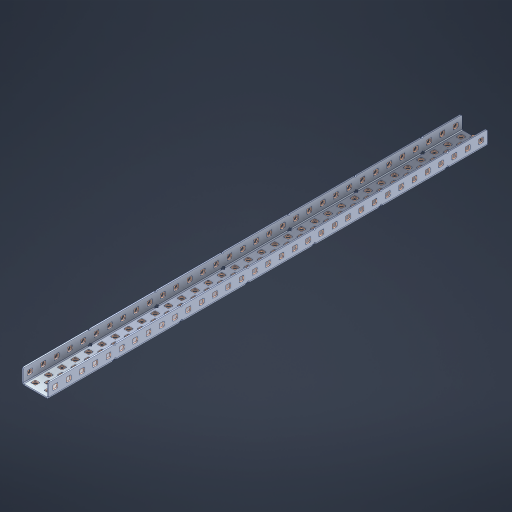
# Autodesk Inventor part: Alu C 1x2x1x35
Saved by Autodesk Inventor 2023 (Build 270158000, 158)
## iProperties
Created: 2022-07-28
Part Number: Alu C 1x2x1x35
Material: Generic
Document SubType Name: Sheet Metal
Designer: ylu12
Density: 1 g/cm^3
Sheet Metal Rule: Default
Appearance: Steel
Author: ylu12
Autodesk Inventor part; units mm, degrees
ref_plane "YZ Plane" through (0, 0, 0) normal (1, 0, 0) x (0, 1, 0)
ref_plane "XZ Plane" through (0, 0, 0) normal (0, 1, 0) x (-1, 0, 0)
sketch "Sketch1" plane through (0, 0, 0) normal (0, 1, 0) x (-1, 0, 0)
  line L0 (-12.7, 0) -> (12.7, 0)
  line L1 (12.7, 0) -> (12.7, -419.1)
  line L2 (12.7, -419.1) -> (-12.7, -419.1)
  line L3 (-12.7, -419.1) -> (-12.7, 0)
  line L4 (12.7, 0) -> (-12.7, -419.1) construction
  point P0 (0, 0)
  point P1 (0, 0)
  dimension "d0" = 25.4
  dimension "d1" = 419.1
  measures "d0" distance of L1.end L2.end
  measures "d1" distance of L0.end L1.end
extrude "Plate1" add sketch "Sketch1" along normal blind 1.1906
sketch "Sketch2" plane through (11.5094, 0, -419.1) normal (1, 0, 0) x (0, 1, 0)
  line L0 (0, 419.1) -> (0, 0)
  line L1 (0, 0) -> (13.8906, 0)
  line L2 (13.8906, 0) -> (13.8906, 419.1)
  line L3 (13.8906, 419.1) -> (0, 419.1)
  constraints: 6 end point, 1 horizontal, 1 perpendicular, 1 vertical
edge flange "Flanges" height 12.7 angle 90 thickness 1.1906 bend radius 0.7937 thickness toward (1, 0, 0) relief tear relief width 1.1906 relief depth 0.5953 corner gap 1.1906 corner form 0 edges at (12.7, 1.1906, -209.55) (-12.7, 1.1906, -209.55) wall of the first edge with corners at (11.5094, 0, 0) (11.5094, 0, -419.1) (11.5094, 13.8906, -419.1) (11.5094, 13.8906, 0)
bend "Bend1"
corner "Corner1"
sketch "Sketch3" plane through (12.7, 1.9844, -419.1) normal (1, 0, 0) x (0, 0, -1)
  line L0 (-414.5534, 7.8676) -> (-410.9466, 7.8676)
  line L1 (-410.4386, 7.3596) -> (-410.4386, 3.7528)
  line L2 (-410.9466, 3.2448) -> (-414.5534, 3.2448)
  line L3 (-415.0614, 3.7528) -> (-415.0614, 7.3596)
  arc A0 (-414.5534, 7.8676) -> (-415.0614, 7.3596) centre (-414.5534, 7.3596) ccw
  arc A1 (-410.4386, 7.3596) -> (-410.9466, 7.8676) centre (-410.9466, 7.3596) ccw
  arc A2 (-410.9466, 3.2448) -> (-410.4386, 3.7528) centre (-410.9466, 3.7528) ccw
  arc A3 (-415.0614, 3.7528) -> (-414.5534, 3.2448) centre (-414.5534, 3.7528) ccw
  line L4 (-419.1, 0) -> (-419.1, 11.9062) construction
  line L5 (-419.1, 11.9062) -> (0, 11.9062) construction
  line L6 (-414.5534, 7.3596) -> (-410.9466, 3.7528) construction
  point P0 (-419.1, -1.9844)
  point P1 (-410.4386, 3.2448)
  point P2 (-415.0614, 3.2448)
  point P3 (-412.75, 5.5562)
  dimension "d16" = 4.6228
  dimension "d17" = 0.508
  dimension "d20" = 6.35
  dimension "d21" = 6.35
  constraints: 10 end point, 8 point on circle, 8 tangent, 4 centre point, 4 point on line, 3 equal radius, 2 parallel, 2 perpendicular, 1 horizontal, 1 midpoint
  measures "d16" distance of point (-410.439, 3.245) point (-415.061, 3.245)
  measures "d17" radius of A0
  measures "d20" distance from line of point (-412.75, 5.556) L4
  measures "d21" distance from line of L5 point (-412.75, 5.556)
extrude "Flange Stamp" cut sketch "Sketch3" against normal blind 1.1906
sketch "Sketch7" plane through (12.7, 1.9844, 0) normal (1, 0, 0) x (0, 0, -1)
  arc A0 (4.5466, 7.8676) -> (4.0386, 7.3596) centre (4.5466, 7.3596) ccw construction
  arc A1 (8.1534, 3.2448) -> (8.6614, 3.7528) centre (8.1534, 3.7528) ccw construction
  circle A2 centre (6.35, 5.5563) radius 2.1844
  line L0 (4.5466, 7.3596) -> (8.1534, 3.7528) construction
  point P0 (0, -1.9844)
  dimension "d46" = 4.3688
  constraints: 2 end point, 1 centre point, 1 midpoint
  measures "d46" diameter of A2
surface extrude "Flange Circle" sketch "Sketch7" against normal up to surface (1.1906 mm away) shown yes curves A2
ref_plane "Flange Pattern Plane" through (12.7, 7.5406, -4.5466) normal (0, 1, 0) x (1, 0, 0)
sketch "Flange Pattern Sketch" plane through (12.7, 7.5406, -4.5466) normal (0, 1, 0) x (1, 0, 0)
  line L0 (0, 3.6068) -> (0, 0) construction
  line L1 (-30.5622, -4.5466) -> (5.5732, -4.5466) construction
  line L2 (0, 0) -> (-1.1906, 0) construction
  point P0 (-12.7, -4.5466)
  point P1 (0, 1.8034)
  point P2 (0, 14.5034)
  point P3 (0, 27.2034)
  point P4 (0, 39.9034)
  point P5 (0, 52.6034)
  point P6 (0, 65.3034)
  point P7 (0, 78.0034)
  point P8 (0, 90.7034)
  point P9 (0, 103.4034)
  point P10 (0, 116.1034)
  point P11 (0, 128.8034)
  point P12 (0, 141.5034)
  point P13 (0, 154.2034)
  point P14 (0, 166.9034)
  point P15 (0, 179.6034)
  point P16 (0, 192.3034)
  point P17 (0, 205.0034)
  point P18 (0, 217.7034)
  point P19 (0, 230.4034)
  point P20 (0, 243.1034)
  point P21 (0, 255.8034)
  point P22 (0, 268.5034)
  point P23 (0, 281.2034)
  point P24 (0, 293.9034)
  point P25 (0, 306.6034)
  point P26 (0, 319.3034)
  point P27 (0, 332.0034)
  point P28 (0, 344.7034)
  point P29 (0, 357.4034)
  point P30 (0, 370.1034)
  point P31 (0, 382.8034)
  point P32 (0, 395.5034)
  point P33 (0, 408.2034)
  point P34 (-25.4, 1.8034)
  point P35 (-25.4, 14.5034)
  point P36 (-25.4, 27.2034)
  point P37 (-25.4, 39.9034)
  point P38 (-25.4, 52.6034)
  point P39 (-25.4, 65.3034)
  point P40 (-25.4, 78.0034)
  point P41 (-25.4, 90.7034)
  point P42 (-25.4, 103.4034)
  point P43 (-25.4, 116.1034)
  point P44 (-25.4, 128.8034)
  point P45 (-25.4, 141.5034)
  point P46 (-25.4, 154.2034)
  point P47 (-25.4, 166.9034)
  point P48 (-25.4, 179.6034)
  point P49 (-25.4, 192.3034)
  point P50 (-25.4, 205.0034)
  point P51 (-25.4, 217.7034)
  point P52 (-25.4, 230.4034)
  point P53 (-25.4, 243.1034)
  point P54 (-25.4, 255.8034)
  point P55 (-25.4, 268.5034)
  point P56 (-25.4, 281.2034)
  point P57 (-25.4, 293.9034)
  point P58 (-25.4, 306.6034)
  point P59 (-25.4, 319.3034)
  point P60 (-25.4, 332.0034)
  point P61 (-25.4, 344.7034)
  point P62 (-25.4, 357.4034)
  point P63 (-25.4, 370.1034)
  point P64 (-25.4, 382.8034)
  point P65 (-25.4, 395.5034)
  point P66 (-25.4, 408.2034)
  dimension "d43" = 25.4
  dimension "d40" = 12.7
  constraints: 1 horizontal, 1 midpoint, 1 vertical, 65 other
  measures "d40" distance of point (0, 1.803) point (0, 14.503)
pattern_sketch "Flange Pattern" of "Flange Circle", "Flange Stamp" from (12.7, 7.5406, -6.35) facing (1, 0, 0) copies at (12.7, 7.5406, -19.05) facing (1, 0, 0) at (12.7, 7.5406, -31.75) facing (1, 0, 0) at (12.7, 7.5406, -44.45) facing (1, 0, 0) at (12.7, 7.5406, -57.15) facing (1, 0, 0) at (12.7, 7.5406, -69.85) facing (1, 0, 0) at (12.7, 7.5406, -82.55) facing (1, 0, 0) at (12.7, 7.5406, -95.25) facing (1, 0, 0) at (12.7, 7.5406, -107.95) facing (1, 0, 0) at (12.7, 7.5406, -120.65) facing (1, 0, 0) at (12.7, 7.5406, -133.35) facing (1, 0, 0) at (12.7, 7.5406, -146.05) facing (1, 0, 0) at (12.7, 7.5406, -158.75) facing (1, 0, 0) at (12.7, 7.5406, -171.45) facing (1, 0, 0) at (12.7, 7.5406, -184.15) facing (1, 0, 0) at (12.7, 7.5406, -196.85) facing (1, 0, 0) at (12.7, 7.5406, -209.55) facing (1, 0, 0) at (12.7, 7.5406, -222.25) facing (1, 0, 0) at (12.7, 7.5406, -234.95) facing (1, 0, 0) at (12.7, 7.5406, -247.65) facing (1, 0, 0) at (12.7, 7.5406, -260.35) facing (1, 0, 0) at (12.7, 7.5406, -273.05) facing (1, 0, 0) at (12.7, 7.5406, -285.75) facing (1, 0, 0) at (12.7, 7.5406, -298.45) facing (1, 0, 0) at (12.7, 7.5406, -311.15) facing (1, 0, 0) at (12.7, 7.5406, -323.85) facing (1, 0, 0) at (12.7, 7.5406, -336.55) facing (1, 0, 0) at (12.7, 7.5406, -349.25) facing (1, 0, 0) at (12.7, 7.5406, -361.95) facing (1, 0, 0) at (12.7, 7.5406, -374.65) facing (1, 0, 0) at (12.7, 7.5406, -387.35) facing (1, 0, 0) at (12.7, 7.5406, -400.05) facing (1, 0, 0) at (12.7, 7.5406, -412.75) facing (1, 0, 0) at (-12.7, 7.5406, -6.35) facing (-1, 0, 0) at (-12.7, 7.5406, -19.05) facing (-1, 0, 0) at (-12.7, 7.5406, -31.75) facing (-1, 0, 0) at (-12.7, 7.5406, -44.45) facing (-1, 0, 0) at (-12.7, 7.5406, -57.15) facing (-1, 0, 0) at (-12.7, 7.5406, -69.85) facing (-1, 0, 0) at (-12.7, 7.5406, -82.55) facing (-1, 0, 0) at (-12.7, 7.5406, -95.25) facing (-1, 0, 0) at (-12.7, 7.5406, -107.95) facing (-1, 0, 0) at (-12.7, 7.5406, -120.65) facing (-1, 0, 0) at (-12.7, 7.5406, -133.35) facing (-1, 0, 0) at (-12.7, 7.5406, -146.05) facing (-1, 0, 0) at (-12.7, 7.5406, -158.75) facing (-1, 0, 0) at (-12.7, 7.5406, -171.45) facing (-1, 0, 0) at (-12.7, 7.5406, -184.15) facing (-1, 0, 0) at (-12.7, 7.5406, -196.85) facing (-1, 0, 0) at (-12.7, 7.5406, -209.55) facing (-1, 0, 0) at (-12.7, 7.5406, -222.25) facing (-1, 0, 0) at (-12.7, 7.5406, -234.95) facing (-1, 0, 0) at (-12.7, 7.5406, -247.65) facing (-1, 0, 0) at (-12.7, 7.5406, -260.35) facing (-1, 0, 0) at (-12.7, 7.5406, -273.05) facing (-1, 0, 0) at (-12.7, 7.5406, -285.75) facing (-1, 0, 0) at (-12.7, 7.5406, -298.45) facing (-1, 0, 0) at (-12.7, 7.5406, -311.15) facing (-1, 0, 0) at (-12.7, 7.5406, -323.85) facing (-1, 0, 0) at (-12.7, 7.5406, -336.55) facing (-1, 0, 0) at (-12.7, 7.5406, -349.25) facing (-1, 0, 0) at (-12.7, 7.5406, -361.95) facing (-1, 0, 0) at (-12.7, 7.5406, -374.65) facing (-1, 0, 0) at (-12.7, 7.5406, -387.35) facing (-1, 0, 0) at (-12.7, 7.5406, -400.05) facing (-1, 0, 0) at (-12.7, 7.5406, -412.75) facing (-1, 0, 0)
sketch "Sketch8" plane through (0, 0, 0) normal (0, -1, 0) x (1, 0, 0)
  line L0 (10.7156, 0) -> (-10.7156, 0) construction
  line L1 (8.1534, -4.0386) -> (4.5466, -4.0386)
  line L2 (4.0386, -4.5466) -> (4.0386, -8.1534)
  line L3 (4.5466, -8.6614) -> (8.1534, -8.6614)
  line L4 (8.6614, -8.1534) -> (8.6614, -4.5466)
  arc A0 (8.6614, -4.5466) -> (8.1534, -4.0386) centre (8.1534, -4.5466) ccw
  arc A1 (8.1534, -8.6614) -> (8.6614, -8.1534) centre (8.1534, -8.1534) ccw
  arc A2 (4.0386, -8.1534) -> (4.5466, -8.6614) centre (4.5466, -8.1534) ccw
  arc A3 (4.5466, -4.0386) -> (4.0386, -4.5466) centre (4.5466, -4.5466) ccw
  line L5 (8.1534, -4.5466) -> (4.5466, -8.1534) construction
  line L6 (12.7, 0) -> (12.7, -419.1) construction
  point P0 (0, 0)
  point P1 (4.0386, -8.6614)
  point P2 (8.6614, -8.6614)
  point P3 (6.35, -6.35)
  dimension "d49" = 4.6228
  dimension "d50" = 0.508
  dimension "d51" = 6.35
  dimension "d52" = 6.35
  constraints: 10 end point, 8 point on circle, 8 tangent, 4 centre point, 4 point on line, 3 equal radius, 2 parallel, 2 perpendicular, 1 horizontal, 1 midpoint
  measures "d49" distance of point (8.661, -8.661) point (4.039, -8.661)
  measures "d50" radius of A0
  measures "d51" distance from line of L6 point (6.35, -6.35)
  measures "d52" distance from line of L0 point (6.35, -6.35)
extrude "Body Stamp" cut sketch "Sketch8" against normal blind 1.1906
sketch "Sketch9" plane through (0, 0, 0) normal (0, -1, 0) x (1, 0, 0)
  arc A0 (8.6614, -4.5466) -> (8.1534, -4.0386) centre (8.1534, -4.5466) ccw construction
  arc A1 (4.0386, -8.1534) -> (4.5466, -8.6614) centre (4.5466, -8.1534) ccw construction
  line L0 (8.1534, -4.5466) -> (4.5466, -8.1534) construction
  circle A2 centre (6.35, -6.35) radius 2.1844
  point P0 (0, 0)
  dimension "d55" = 4.3688
  constraints: 2 end point, 1 centre point, 1 midpoint
  measures "d55" diameter of A2
surface extrude "Body Circle" sketch "Sketch9" against normal up to surface (1.1906 mm away) shown yes curves A2
pattern_sketch "Body Pattern" of "Body Stamp", "Body Circle" from (6.35, 0, -6.35) copies at (6.35, 0, -19.05) at (6.35, 0, -31.75) at (6.35, 0, -44.45) at (6.35, 0, -57.15) at (6.35, 0, -69.85) at (6.35, 0, -82.55) at (6.35, 0, -95.25) at (6.35, 0, -107.95) at (6.35, 0, -120.65) at (6.35, 0, -133.35) at (6.35, 0, -146.05) at (6.35, 0, -158.75) at (6.35, 0, -171.45) at (6.35, 0, -184.15) at (6.35, 0, -196.85) at (6.35, 0, -209.55) at (6.35, 0, -222.25) at (6.35, 0, -234.95) at (6.35, 0, -247.65) at (6.35, 0, -260.35) at (6.35, 0, -273.05) at (6.35, 0, -285.75) at (6.35, 0, -298.45) at (6.35, 0, -311.15) at (6.35, 0, -323.85) at (6.35, 0, -336.55) at (6.35, 0, -349.25) at (6.35, 0, -361.95) at (6.35, 0, -374.65) at (6.35, 0, -387.35) at (6.35, 0, -400.05) at (6.35, 0, -412.75) at (-6.35, 0, -6.35) at (-6.35, 0, -19.05) at (-6.35, 0, -31.75) at (-6.35, 0, -44.45) at (-6.35, 0, -57.15) at (-6.35, 0, -69.85) at (-6.35, 0, -82.55) at (-6.35, 0, -95.25) at (-6.35, 0, -107.95) at (-6.35, 0, -120.65) at (-6.35, 0, -133.35) at (-6.35, 0, -146.05) at (-6.35, 0, -158.75) at (-6.35, 0, -171.45) at (-6.35, 0, -184.15) at (-6.35, 0, -196.85) at (-6.35, 0, -209.55) at (-6.35, 0, -222.25) at (-6.35, 0, -234.95) at (-6.35, 0, -247.65) at (-6.35, 0, -260.35) at (-6.35, 0, -273.05) at (-6.35, 0, -285.75) at (-6.35, 0, -298.45) at (-6.35, 0, -311.15) at (-6.35, 0, -323.85) at (-6.35, 0, -336.55) at (-6.35, 0, -349.25) at (-6.35, 0, -361.95) at (-6.35, 0, -374.65) at (-6.35, 0, -387.35) at (-6.35, 0, -400.05) at (-6.35, 0, -412.75)
sketch "Sketch15" plane through (0, 0, 0) normal (0, -1, 0) x (1, 0, 0)
  line L0 (10.7156, 0) -> (-10.7156, 0) construction
  line L1 (1.8034, -10.3886) -> (-1.8034, -10.3886)
  line L2 (-2.3114, -10.8966) -> (-2.3114, -14.5034)
  line L3 (-1.8034, -15.0114) -> (1.8034, -15.0114)
  line L4 (2.3114, -14.5034) -> (2.3114, -10.8966)
  arc A0 (2.3114, -10.8966) -> (1.8034, -10.3886) centre (1.8034, -10.8966) ccw
  arc A1 (1.8034, -15.0114) -> (2.3114, -14.5034) centre (1.8034, -14.5034) ccw
  arc A2 (-1.8034, -10.3886) -> (-2.3114, -10.8966) centre (-1.8034, -10.8966) ccw
  arc A3 (-2.3114, -14.5034) -> (-1.8034, -15.0114) centre (-1.8034, -14.5034) ccw
  line L5 (1.8034, -10.8966) -> (-1.8034, -14.5034) construction
  line L6 (12.7, 0) -> (12.7, -419.1) construction
  point P0 (0, 0)
  point P1 (-2.3114, -15.0114)
  point P2 (2.3114, -15.0114)
  point P3 (0, -12.7)
  dimension "d106" = 4.6228
  dimension "d107" = 0.508
  dimension "d108" = 12.7
  dimension "d109" = 12.7
  constraints: 10 end point, 8 point on circle, 8 tangent, 4 centre point, 4 point on line, 3 equal radius, 2 parallel, 2 perpendicular, 1 horizontal, 1 midpoint
  measures "d106" distance of point (2.311, -15.011) point (-2.311, -15.011)
  measures "d107" radius of A0
  measures "d108" distance from line of L0 point (0, -12.7)
  measures "d109" distance from line of L6 point (0, -12.7)
extrude "Center Stamp" cut sketch "Sketch15" against normal blind 1.1906
sketch "Sketch16" plane through (0, 0, 0) normal (0, -1, 0) x (1, 0, 0)
  circle A0 centre (0, -12.7) radius 2.1844
  line L0 (10.7156, 0) -> (-10.7156, 0) construction
  line L1 (12.7, 0) -> (12.7, -419.1) construction
  point P0 (0, 0)
  dimension "d112" = 4.3688
  dimension "d118" = 12.7
  dimension "d119" = 12.7
  constraints: 1 centre point
  measures "d112" diameter of A0
  measures "d118" distance from line of L0 A0.centre
  measures "d119" distance from line of L1 A0.centre
surface extrude "Center Circle" sketch "Sketch16" against normal up to surface (1.1906 mm away) shown yes curves A0
pattern_linear "Center Pattern" count 33 spacing 12.7 along (0, 0, -1) of "Center Circle", "Center Stamp"
sketch "Arc Length" plane through (11.5094, 1.9844, 0) normal (0, 0, 1) x (1, 0, 0)
  line L0 (0, 0) -> (1.1906, 0) construction
  arc A0 (-0.7938, -0.7938) -> (0, 0) centre (-0.7938, 0) ccw construction
  line L1 (-0.7938, -1.9844) -> (-0.7938, -0.7938) construction
  arc A1 (-0.7938, -1.9844) -> (1.1906, 0) centre (-0.7938, 0) ccw construction
  point P0 (-11.5094, -1.9844)
  dimension "d85" = 3.117
  dimension "d92" = 1.2468
sketch "Sketch13" plane through (12.7, 13.8906, 0) normal (1, 0, 0) x (0, 0, -1)
  line L0 (0, 0) -> (419.1, 0) construction
  line L1 (62.4078, 0) -> (63.4238, -1.016)
  line L2 (63.4238, -1.016) -> (64.4398, 0)
  line L3 (62.4078, 0) -> (64.4398, 0)
  line L4 (419.1, -11.9062) -> (0, -11.9063) construction
  line L5 (63.4238, -10.8903) -> (61.3168, -12.9972)
  line L6 (61.3168, -12.9972) -> (63.4238, -15.1042)
  line L7 (63.4238, -15.1042) -> (65.5308, -12.9972)
  line L8 (65.5308, -12.9972) -> (63.4238, -10.8903)
  line L9 (63.4238, -10.8903) -> (63.4238, -15.1042) construction
  line L10 (63.4238, -1.016) -> (63.4238, -10.8903) construction
  line L11 (0, -11.9063) -> (419.1, -11.9062) construction
  point P0 (0, -13.8906)
  dimension "d86" = 4.2139
  dimension "d88" = 1.016
  dimension "d91" = 1.016
  dimension "d102" = 63.4238
  constraints: 19 end point, 6 perpendicular, 2 point on line, 2 vertical, 1 collinear
  measures "d86" distance of L5.start L6.end
  measures "d88" distance from line of L0 L1.end
  measures "d91" distance from line of L5.start L11
  measures "d102" distance from line of L0.start L10
cut across bends "Notch" sketch "Sketch13" k factor 0.44
mirror "Notch Mirror" about plane through (0, 0, 0) normal (1, 0, 0) of "Notch"
pattern_linear "Notch Pattern" count 6 spacing 63.5 along (0, 0, -1) of "Notch", "Notch Mirror"
chamfer "End Chamfer" distance 1.016 angle 45 4 edges at (-12.1047, 13.8906, -419.1) (12.1047, 13.8906, -419.1) (-12.1047, 13.8906, 0) (12.1047, 13.8906, 0)
sketch "Sketch14" plane through (-12.7, 1.9844, 25.4) normal (1, 0, 0) x (0, 0, -1)
  line L0 (25.4, 11.9062) -> (444.5, 11.9062) construction
  line L1 (25.4, 0) -> (25.4, 11.9062) construction
  line L2 (25.4, -1.9844) -> (444.5, -1.9844) construction
  line L3 (25.4, 11.9062) -> (444.5, 11.9062)
  line L4 (444.5, 11.9062) -> (444.5, -1.9844)
  line L5 (444.5, -1.9844) -> (25.4, -1.9844)
  line L6 (25.4, -1.9844) -> (25.4, 11.9062)
  point P0 (87.8078, 11.9062)
  point P1 (26.416, 11.9062)
  point P2 (25.4, 10.8902)
  point P3 (407.4521, -1.9844)
  point P4 (443.484, 11.9062)
  point P5 (280.3398, 11.9062)
  point P6 (341.8078, 11.9062)
  constraints: 8 end point, 2 collinear, 2 parallel, 1 horizontal, 1 perpendicular
extrude "Half Cut" [suppressed]
sketch "Body Pattern Sketch" plane through (0, 0, 0) normal (0, -1, 0) x (1, 0, 0)
  line L0 (10.7156, 0) -> (-10.7156, 0) construction
  line L1 (12.7, 0) -> (12.7, -419.1) construction
  point P0 (0, 0)
  point P1 (6.35, -6.35)
  point P2 (6.35, -19.05)
  point P3 (6.35, -31.75)
  point P4 (6.35, -44.45)
  point P5 (6.35, -57.15)
  point P6 (6.35, -69.85)
  point P7 (6.35, -82.55)
  point P8 (6.35, -95.25)
  point P9 (6.35, -107.95)
  point P10 (6.35, -120.65)
  point P11 (6.35, -133.35)
  point P12 (6.35, -146.05)
  point P13 (6.35, -158.75)
  point P14 (6.35, -171.45)
  point P15 (6.35, -184.15)
  point P16 (6.35, -196.85)
  point P17 (6.35, -209.55)
  point P18 (6.35, -222.25)
  point P19 (6.35, -234.95)
  point P20 (6.35, -247.65)
  point P21 (6.35, -260.35)
  point P22 (6.35, -273.05)
  point P23 (6.35, -285.75)
  point P24 (6.35, -298.45)
  point P25 (6.35, -311.15)
  point P26 (6.35, -323.85)
  point P27 (6.35, -336.55)
  point P28 (6.35, -349.25)
  point P29 (6.35, -361.95)
  point P30 (6.35, -374.65)
  point P31 (6.35, -387.35)
  point P32 (6.35, -400.05)
  point P33 (6.35, -412.75)
  point P34 (-6.35, -6.35)
  point P35 (-6.35, -19.05)
  point P36 (-6.35, -31.75)
  point P37 (-6.35, -44.45)
  point P38 (-6.35, -57.15)
  point P39 (-6.35, -69.85)
  point P40 (-6.35, -82.55)
  point P41 (-6.35, -95.25)
  point P42 (-6.35, -107.95)
  point P43 (-6.35, -120.65)
  point P44 (-6.35, -133.35)
  point P45 (-6.35, -146.05)
  point P46 (-6.35, -158.75)
  point P47 (-6.35, -171.45)
  point P48 (-6.35, -184.15)
  point P49 (-6.35, -196.85)
  point P50 (-6.35, -209.55)
  point P51 (-6.35, -222.25)
  point P52 (-6.35, -234.95)
  point P53 (-6.35, -247.65)
  point P54 (-6.35, -260.35)
  point P55 (-6.35, -273.05)
  point P56 (-6.35, -285.75)
  point P57 (-6.35, -298.45)
  point P58 (-6.35, -311.15)
  point P59 (-6.35, -323.85)
  point P60 (-6.35, -336.55)
  point P61 (-6.35, -349.25)
  point P62 (-6.35, -361.95)
  point P63 (-6.35, -374.65)
  point P64 (-6.35, -387.35)
  point P65 (-6.35, -400.05)
  point P66 (-6.35, -412.75)
  dimension "d62" = 12.7
  dimension "d65" = 12.7
  dimension "d58" = 6.35
  dimension "d99" = 6.35
  constraints: 1 horizontal, 1 vertical, 65 other
  measures "d58" distance from line of L1 point (6.35, -6.35)
  measures "d99" distance from line of L0 point (6.35, -6.35)
equation "\"d1\" = 12.7 * Length"
equation "\"d18\" = Thickness"
equation "\"d53\" = Thickness"
equation "\"d89\" = Thickness"
equation "\"d2\" = Thickness"
equation "\"d3\" = BendReliefWidth"
equation "\"d4\" = BendReliefDepth"
equation "\"d5\" = MinimumRemnant"
equation "\"d6\" = TransitionRadius"
equation "\"d10\" = CornerReliefSize"
equation "\"d11\" = GapSize"
equation "\"d12\" = JacobiRadiusSize"
equation "\"BendRadius\" = Thickness"
equation "\"BendReliefWidth\" = Thickness"
equation "\"BendReliefDepth\" = 0.5 * Thickness"
equation "\"CornerReliefSize\" = 4 * Thickness"
equation "\"MinimumRemnant\" = 2 * Thickness"
equation "\"TransitionRadius\" = BendRadius"
equation "\"JacobiRadiusSize\" = BendRadius"
equation "\"GapSize\" = Thickness"
equation "\"Length\" = 33"
equation "\"Thickness\" = 1.190625"
body "Solid1"
body "Srf1"
body "Srf2"
body "Srf91"
body "Srf92"
body "Srf786"
body "Srf823"
body "Srf824"
body "Srf825"
body "Srf826"
body "Srf827"
body "Srf828"
body "Srf829"
body "Srf856"
body "Srf857"
body "Srf858"
body "Srf859"
body "Srf860"
body "Srf861"
body "Srf862"
body "Srf889"
body "Srf890"
body "Srf891"
body "Srf892"
body "Srf893"
body "Srf894"
body "Srf895"
body "Srf896"
body "Srf922"
body "Srf923"
body "Srf924"
body "Srf925"
body "Srf926"
body "Srf959"
body "Srf960"
body "Srf961"
body "Srf962"
body "Srf963"
body "Srf996"
body "Srf997"
body "Srf998"
body "Srf999"
body "Srf1000"
body "Srf1143"
body "Srf1144"
body "Srf1145"
body "Srf1146"
body "Srf1147"
body "Srf1148"
body "Srf1149"
body "Srf1150"
body "Srf1151"
body "Srf1152"
body "Srf1153"
body "Srf1154"
body "Srf1155"
body "Srf1156"
body "Srf1157"
body "Srf1158"
body "Srf1159"
body "Srf1160"
body "Srf1161"
body "Srf1162"
body "Srf1163"
body "Srf1164"
body "Srf1165"
body "Srf1166"
body "Srf1167"
body "Srf1168"
body "Srf1169"
body "Srf1170"
body "Srf1171"
body "Srf1172"
body "Srf1173"
body "Srf1174"
body "Srf1175"
body "Srf1176"
body "Srf1177"
body "Srf1178"
body "Srf1179"
body "Srf1180"
body "Srf1181"
body "Srf1182"
body "Srf1183"
body "Srf1184"
body "Srf1185"
body "Srf1186"
body "Srf1187"
body "Srf1188"
body "Srf1189"
body "Srf1190"
body "Srf1191"
body "Srf1192"
body "Srf1193"
body "Srf1194"
body "Srf1199"
body "Srf1200"
body "Srf1201"
body "Srf1202"
body "Srf1203"
body "Srf1204"
body "Srf1205"
body "Srf1206"
body "Srf1207"
body "Srf1208"
body "Srf1209"
body "Srf1210"
body "Srf1211"
body "Srf1212"
body "Srf1213"
body "Srf1214"
body "Srf1215"
body "Srf1216"
body "Srf1217"
body "Srf1218"
body "Srf1219"
body "Srf1220"
body "Srf1221"
body "Srf1222"
body "Srf1223"
body "Srf1224"
body "Srf1225"
body "Srf1226" dims "d40" = 12.7, "d43" = 25.4
body "Srf1227"
body "Srf1228"
body "Srf1229"
body "Srf1230"
body "Srf1231"
body "Srf1232"
body "Srf1233"
body "Srf1234"
body "Srf1235"
body "Srf1236"
body "Srf1237"
body "Srf1238"
body "Srf1239"
body "Srf1240"
body "Srf1241"
body "Srf1242"
body "Srf1243"
body "Srf1244"
body "Srf1245"
body "Srf1246"
body "Srf1247"
body "Srf1248"
body "Srf1249"
body "Srf1250"
body "Srf1255"
body "Srf1256"
body "Srf1257"
body "Srf1258"
body "Srf1259"
body "Srf1260"
body "Srf1261"
body "Srf1262"
body "Srf1263"
body "Srf1264"
body "Srf1265"
body "Srf1266"
body "Srf1267"
body "Srf1268"
body "Srf1269"
body "Srf1270"
body "Srf1271"
body "Srf1272"
body "Srf1273"
